Autodesk Fusion 360 part; units mm, degrees
(part 3 of 4)
  spline S213 degree 3 poles (-242.4, 76) (-242.5104, 76) (-242.6, 76.0895) (-242.6, 76.2) knots 6 6 6 6 7 7 7 7
  line L339 (-242.6, 76.2) -> (-242.6, 89.8)
  spline S214 degree 3 poles (-242.6, 89.8) (-242.6, 89.9104) (-242.5104, 90) (-242.4, 90) knots 0 0 0 0 1 1 1 1
  line L340 (-242.4, 90) -> (-228.8, 90)
  spline S215 degree 3 poles (-228.8, 90) (-228.6896, 90) (-228.6, 89.9104) (-228.6, 89.8) knots 2 2 2 2 3 3 3 3
  line L341 (-228.6, 89.8) -> (-228.6, 76.2)
  spline S216 degree 3 poles (-228.6, 76.2) (-228.6, 76.0895) (-228.6896, 76) (-228.8, 76) knots 4 4 4 4 5 5 5 5
  line L342 (-228.8, 76) -> (-242.4, 76)
  spline S217 degree 3 poles (-240.705, 70.95) (-240.5946, 70.95) (-240.505, 70.8604) (-240.505, 70.75) knots 6 6 6 6 7 7 7 7
  line L343 (-240.505, 70.75) -> (-240.505, 57.15)
  spline S218 degree 3 poles (-240.505, 57.15) (-240.505, 57.0395) (-240.5946, 56.95) (-240.705, 56.95) knots 0 0 0 0 1 1 1 1
  line L344 (-240.705, 56.95) -> (-254.3051, 56.95)
  spline S219 degree 3 poles (-254.3051, 56.95) (-254.4155, 56.95) (-254.5051, 57.0395) (-254.5051, 57.15) knots 2 2 2 2 3 3 3 3
  line L345 (-254.5051, 57.15) -> (-254.5051, 70.75)
  spline S220 degree 3 poles (-254.5051, 70.75) (-254.5051, 70.8604) (-254.4155, 70.95) (-254.3051, 70.95) knots 4 4 4 4 5 5 5 5
  line L346 (-254.3051, 70.95) -> (-240.705, 70.95)
  spline S221 degree 3 poles (-157.3601, 70.95) (-157.2497, 70.95) (-157.1601, 70.8604) (-157.1601, 70.75) knots 6 6 6 6 7 7 7 7
  line L347 (-157.1601, 70.75) -> (-157.1601, 57.15)
  spline S222 degree 3 poles (-157.1601, 57.15) (-157.1601, 57.0395) (-157.2497, 56.95) (-157.3601, 56.95) knots 0 0 0 0 1 1 1 1
  line L348 (-157.3601, 56.95) -> (-170.9601, 56.95)
  spline S223 degree 3 poles (-170.9601, 56.95) (-171.0705, 56.95) (-171.1601, 57.0395) (-171.1601, 57.15) knots 2 2 2 2 3 3 3 3
  line L349 (-171.1601, 57.15) -> (-171.1601, 70.75)
  spline S224 degree 3 poles (-171.1601, 70.75) (-171.1601, 70.8604) (-171.0705, 70.95) (-170.9601, 70.95) knots 4 4 4 4 5 5 5 5
  line L350 (-170.9601, 70.95) -> (-157.3601, 70.95)
  spline S225 degree 3 poles (-180.6801, 51.7) (-180.6801, 51.8104) (-180.5905, 51.9) (-180.4801, 51.9) knots 6 6 6 6 7 7 7 7
  line L351 (-180.4801, 51.9) -> (-166.8801, 51.9)
  spline S226 degree 3 poles (-166.8801, 51.9) (-166.7697, 51.9) (-166.6801, 51.8104) (-166.6801, 51.7) knots 0 0 0 0 1 1 1 1
  line L352 (-166.6801, 51.7) -> (-166.6801, 38.1)
  spline S227 degree 3 poles (-166.6801, 38.1) (-166.6801, 37.9895) (-166.7697, 37.9) (-166.8801, 37.9) knots 2 2 2 2 3 3 3 3
  line L353 (-166.8801, 37.9) -> (-180.4801, 37.9)
  spline S228 degree 3 poles (-180.4801, 37.9) (-180.5905, 37.9) (-180.6801, 37.9895) (-180.6801, 38.1) knots 4 4 4 4 5 5 5 5
  line L354 (-180.6801, 38.1) -> (-180.6801, 51.7)
  spline S229 degree 3 poles (-152.6, 13.8) (-152.4896, 13.8) (-152.4, 13.7104) (-152.4, 13.6) knots 6 6 6 6 7 7 7 7
  line L355 (-152.4, 13.6) -> (-152.4, 0)
  spline S230 degree 3 poles (-152.4, 0) (-152.4, -0.1105) (-152.4896, -0.2) (-152.6, -0.2) knots 0 0 0 0 1 1 1 1
  line L356 (-152.6, -0.2) -> (-166.2, -0.2)
  spline S231 degree 3 poles (-166.2, -0.2) (-166.3104, -0.2) (-166.4, -0.1105) (-166.4, 0) knots 2 2 2 2 3 3 3 3
  line L357 (-166.4, 0) -> (-166.4, 13.6)
  spline S232 degree 3 poles (-166.4, 13.6) (-166.4, 13.7104) (-166.3104, 13.8) (-166.2, 13.8) knots 4 4 4 4 5 5 5 5
  line L358 (-166.2, 13.8) -> (-152.6, 13.8)
  line L359 (-156.68, 32.85) -> (-143.0802, 32.85)
  spline S233 degree 3 poles (-143.0802, 32.85) (-142.9696, 32.85) (-142.88, 32.7604) (-142.88, 32.65) knots 7 7 7 7 8 8 8 8
  line L360 (-142.88, 32.65) -> (-142.88, 19.05)
  spline S234 degree 3 poles (-142.88, 19.05) (-142.88, 18.9395) (-142.9696, 18.85) (-143.0802, 18.85) knots 1 1 1 1 2 2 2 2
  line L361 (-143.0802, 18.85) -> (-156.68, 18.85)
  spline S235 degree 3 poles (-156.68, 18.85) (-156.7906, 18.85) (-156.88, 18.9395) (-156.88, 19.05) knots 3 3 3 3 4 4 4 4
  line L362 (-156.88, 19.05) -> (-156.88, 32.65)
  spline S236 degree 3 poles (-156.88, 32.65) (-156.88, 32.7604) (-156.7906, 32.85) (-156.68, 32.85) knots 5 5 5 5 6 6 6 6
  line L363 (-118.58, 32.85) -> (-104.9802, 32.85)
  spline S237 degree 3 poles (-104.9802, 32.85) (-104.8696, 32.85) (-104.78, 32.7604) (-104.78, 32.65) knots 7 7 7 7 8 8 8 8
  line L364 (-104.78, 32.65) -> (-104.78, 19.05)
  spline S238 degree 3 poles (-104.78, 19.05) (-104.78, 18.9395) (-104.8696, 18.85) (-104.9802, 18.85) knots 1 1 1 1 2 2 2 2
  line L365 (-104.9802, 18.85) -> (-118.58, 18.85)
  spline S239 degree 3 poles (-118.58, 18.85) (-118.6906, 18.85) (-118.78, 18.9395) (-118.78, 19.05) knots 3 3 3 3 4 4 4 4
  line L366 (-118.78, 19.05) -> (-118.78, 32.65)
  spline S240 degree 3 poles (-118.78, 32.65) (-118.78, 32.7604) (-118.6906, 32.85) (-118.58, 32.85) knots 5 5 5 5 6 6 6 6
  line L367 (-175.73, 32.85) -> (-162.1302, 32.85)
  spline S241 degree 3 poles (-162.1302, 32.85) (-162.0196, 32.85) (-161.93, 32.7604) (-161.93, 32.65) knots 7 7 7 7 8 8 8 8
  line L368 (-161.93, 32.65) -> (-161.93, 19.05)
  spline S242 degree 3 poles (-161.93, 19.05) (-161.93, 18.9395) (-162.0196, 18.85) (-162.1302, 18.85) knots 1 1 1 1 2 2 2 2
  line L369 (-162.1302, 18.85) -> (-175.73, 18.85)
  spline S243 degree 3 poles (-175.73, 18.85) (-175.8406, 18.85) (-175.93, 18.9395) (-175.93, 19.05) knots 3 3 3 3 4 4 4 4
  line L370 (-175.93, 19.05) -> (-175.93, 32.65)
  spline S244 degree 3 poles (-175.93, 32.65) (-175.93, 32.7604) (-175.8406, 32.85) (-175.73, 32.85) knots 5 5 5 5 6 6 6 6
  line L371 (-99.53, 32.85) -> (-85.9302, 32.85)
  spline S245 degree 3 poles (-85.9302, 32.85) (-85.8196, 32.85) (-85.73, 32.7604) (-85.73, 32.65) knots 7 7 7 7 8 8 8 8
  line L372 (-85.73, 32.65) -> (-85.73, 19.05)
  spline S246 degree 3 poles (-85.73, 19.05) (-85.73, 18.9395) (-85.8196, 18.85) (-85.9302, 18.85) knots 1 1 1 1 2 2 2 2
  line L373 (-85.9302, 18.85) -> (-99.53, 18.85)
  spline S247 degree 3 poles (-99.53, 18.85) (-99.6406, 18.85) (-99.73, 18.9395) (-99.73, 19.05) knots 3 3 3 3 4 4 4 4
  line L374 (-99.73, 19.05) -> (-99.73, 32.65)
  spline S248 degree 3 poles (-99.73, 32.65) (-99.73, 32.7604) (-99.6406, 32.85) (-99.53, 32.85) knots 5 5 5 5 6 6 6 6
  spline S249 degree 3 poles (-138.3101, 70.95) (-138.1997, 70.95) (-138.1101, 70.8604) (-138.1101, 70.75) knots 6 6 6 6 7 7 7 7
  line L375 (-138.1101, 70.75) -> (-138.1101, 57.15)
  spline S250 degree 3 poles (-138.1101, 57.15) (-138.1101, 57.0395) (-138.1997, 56.95) (-138.3101, 56.95) knots 0 0 0 0 1 1 1 1
  line L376 (-138.3101, 56.95) -> (-151.9101, 56.95)
  spline S251 degree 3 poles (-151.9101, 56.95) (-152.0205, 56.95) (-152.1101, 57.0395) (-152.1101, 57.15) knots 2 2 2 2 3 3 3 3
  line L377 (-152.1101, 57.15) -> (-152.1101, 70.75)
  spline S252 degree 3 poles (-152.1101, 70.75) (-152.1101, 70.8604) (-152.0205, 70.95) (-151.9101, 70.95) knots 4 4 4 4 5 5 5 5
  line L378 (-151.9101, 70.95) -> (-138.3101, 70.95)
  spline S253 degree 3 poles (-52.5801, 51.9) (-52.4697, 51.9) (-52.3801, 51.8104) (-52.3801, 51.7) knots 6 6 6 6 7 7 7 7
  line L379 (-52.3801, 51.7) -> (-52.3801, 38.1)
  spline S254 degree 3 poles (-52.3801, 38.1) (-52.3801, 37.9895) (-52.4697, 37.9) (-52.5801, 37.9) knots 0 0 0 0 1 1 1 1
  line L380 (-52.5801, 37.9) -> (-66.1801, 37.9)
  spline S255 degree 3 poles (-66.1801, 37.9) (-66.2905, 37.9) (-66.3801, 37.9895) (-66.3801, 38.1) knots 2 2 2 2 3 3 3 3
  line L381 (-66.3801, 38.1) -> (-66.3801, 51.7)
  spline S256 degree 3 poles (-66.3801, 51.7) (-66.3801, 51.8104) (-66.2905, 51.9) (-66.1801, 51.9) knots 4 4 4 4 5 5 5 5
  line L382 (-66.1801, 51.9) -> (-52.5801, 51.9)
  line L383 (-80.48, 32.85) -> (-66.8802, 32.85)
  spline S257 degree 3 poles (-66.8802, 32.85) (-66.7696, 32.85) (-66.68, 32.7604) (-66.68, 32.65) knots 7 7 7 7 8 8 8 8
  line L384 (-66.68, 32.65) -> (-66.68, 19.05)
  spline S258 degree 3 poles (-66.68, 19.05) (-66.68, 18.9395) (-66.7696, 18.85) (-66.8802, 18.85) knots 1 1 1 1 2 2 2 2
  line L385 (-66.8802, 18.85) -> (-80.48, 18.85)
  spline S259 degree 3 poles (-80.48, 18.85) (-80.5906, 18.85) (-80.68, 18.9395) (-80.68, 19.05) knots 3 3 3 3 4 4 4 4
  line L386 (-80.68, 19.05) -> (-80.68, 32.65)
  spline S260 degree 3 poles (-80.68, 32.65) (-80.68, 32.7604) (-80.5906, 32.85) (-80.48, 32.85) knots 5 5 5 5 6 6 6 6
  spline S261 degree 3 poles (-114.5, 13.8) (-114.3896, 13.8) (-114.3, 13.7104) (-114.3, 13.6) knots 6 6 6 6 7 7 7 7
  line L387 (-114.3, 13.6) -> (-114.3, 0)
  spline S262 degree 3 poles (-114.3, 0) (-114.3, -0.1105) (-114.3896, -0.2) (-114.5, -0.2) knots 0 0 0 0 1 1 1 1
  line L388 (-114.5, -0.2) -> (-128.1, -0.2)
  spline S263 degree 3 poles (-128.1, -0.2) (-128.2104, -0.2) (-128.3, -0.1105) (-128.3, 0) knots 2 2 2 2 3 3 3 3
  line L389 (-128.3, 0) -> (-128.3, 13.6)
  spline S264 degree 3 poles (-128.3, 13.6) (-128.3, 13.7104) (-128.2104, 13.8) (-128.1, 13.8) knots 4 4 4 4 5 5 5 5
  line L390 (-128.1, 13.8) -> (-114.5, 13.8)
  spline S265 degree 3 poles (-214.03, 32.65) (-214.03, 32.7604) (-213.9406, 32.85) (-213.83, 32.85) knots 6 6 6 6 7 7 7 7
  line L391 (-213.83, 32.85) -> (-200.2302, 32.85)
  spline S266 degree 3 poles (-200.2302, 32.85) (-200.1196, 32.85) (-200.03, 32.7604) (-200.03, 32.65) knots 0 0 0 0 1 1 1 1
  line L392 (-200.03, 32.65) -> (-200.03, 19.05)
  spline S267 degree 3 poles (-200.03, 19.05) (-200.03, 18.9395) (-200.1196, 18.85) (-200.2302, 18.85) knots 2 2 2 2 3 3 3 3
  line L393 (-200.2302, 18.85) -> (-213.83, 18.85)
  spline S268 degree 3 poles (-213.83, 18.85) (-213.9406, 18.85) (-214.03, 18.9395) (-214.03, 19.05) knots 4 4 4 4 5 5 5 5
  line L394 (-214.03, 19.05) -> (-214.03, 32.65)
  spline S269 degree 3 poles (-171.65, 13.8) (-171.5396, 13.8) (-171.45, 13.7104) (-171.45, 13.6) knots 6 6 6 6 7 7 7 7
  line L395 (-171.45, 13.6) -> (-171.45, 0)
  spline S270 degree 3 poles (-171.45, 0) (-171.45, -0.1105) (-171.5396, -0.2) (-171.65, -0.2) knots 0 0 0 0 1 1 1 1
  line L396 (-171.65, -0.2) -> (-185.25, -0.2)
  spline S271 degree 3 poles (-185.25, -0.2) (-185.3604, -0.2) (-185.45, -0.1105) (-185.45, 0) knots 2 2 2 2 3 3 3 3
  line L397 (-185.45, 0) -> (-185.45, 13.6)
  spline S272 degree 3 poles (-185.45, 13.6) (-185.45, 13.7104) (-185.3604, 13.8) (-185.25, 13.8) knots 4 4 4 4 5 5 5 5
  line L398 (-185.25, 13.8) -> (-171.65, 13.8)
  arc A8 (13, 95) -> (5, 103) centre (5, 95) ccw
  line L399 (5, 103) -> (-304.75, 103)
  arc A9 (-304.75, 103) -> (-312.75, 95) centre (-304.75, 95) ccw
  line L400 (-312.75, 95) -> (-312.75, -5.2)
  arc A10 (-312.75, -5.2) -> (-304.75, -13.2) centre (-304.75, -5.2) ccw
  line L401 (-304.75, -13.2) -> (5, -13.2)
  arc A11 (5, -13.2) -> (13, -5.2) centre (5, -5.2) ccw
  line L402 (13, -5.2) -> (13, 95)
  line L403 (3, -3.2) -> (-302.75, -3.2)
  line L404 (-302.75, -3.2) -> (-302.75, 93)
  line L405 (-302.75, 93) -> (3, 93)
  line L406 (3, 93) -> (3, -3.2)
  dimension "d354" = 3
  dimension "d355" = 3
  dimension "d356" = 3
  dimension "d358" = 3
  constraint horizontal L403
  constraint vertical L404
  constraint horizontal L405
  constraint vertical L406
  measures "d354" distance of L323 L404
  measures "d355" distance of L326 L403
  measures "d356" distance of L45 L405
  measures "d358" distance of L33 L406
extrude "Extrude2" add sketch "led-plate" along normal blind 3 separate body contours A8 L399 A9 L400 A10 L401 A11 L402 makes body 2 in component "led-plate"
sketch "top-plate" plane through (0, 0, 4.5) normal (0, 0, 1) x (-1, 0, 0) in component "top-plate"
  circle A0 centre (-228.8125, 98) radius 1
  circle A1 centre (-70.9375, 98) radius 1
  circle A2 centre (-70.9375, -8.2) radius 1
  circle A3 centre (-307.75, -8.2) radius 1
  circle A4 centre (-307.75, 98) radius 1
  circle A5 centre (8, 98) radius 1
  circle A6 centre (-228.8125, -8.2) radius 1
  circle A7 centre (8, -8.2) radius 1
  arc A8 (13, 95) -> (5, 103) centre (5, 95) ccw
  line L0 (5, 103) -> (-304.75, 103)
  arc A9 (-304.75, 103) -> (-312.75, 95) centre (-304.75, 95) ccw
  line L1 (-312.75, 95) -> (-312.75, -5.2)
  arc A10 (-312.75, -5.2) -> (-304.75, -13.2) centre (-304.75, -5.2) ccw
  line L2 (-304.75, -13.2) -> (5, -13.2)
  arc A11 (5, -13.2) -> (13, -5.2) centre (5, -5.2) ccw
  line L3 (13, -5.2) -> (13, 95)
  line L4 (8, -8.2) -> (8, 98) construction
  line L5 (8, 10.7161) -> (8, 79.0839)
  line L6 (13, -5.2) -> (13, 4.8)
  line L7 (13, 95) -> (13, 85)
  arc A12 (8, 10.7161) -> (10.5, 7.758) centre (11, 10.7161) ccw
  arc A13 (10.5, 82.042) -> (13, 85) centre (10, 85) ccw
  arc A14 (13, 4.8) -> (10.5, 7.758) centre (10, 4.8) ccw
  arc A15 (10.5, 82.042) -> (8, 79.0839) centre (11, 79.0839) ccw
  line L8 (-307.75, -8.2) -> (-307.75, 98) construction
  line L9 (-312.75, -5.2) -> (-312.75, 4.8)
  line L10 (-312.75, 95) -> (-312.75, 85)
  line L11 (-307.75, 79.0839) -> (-307.75, 10.7161)
  arc A16 (-310.25, 7.758) -> (-312.75, 4.8) centre (-309.75, 4.8) ccw
  arc A17 (-310.25, 7.758) -> (-307.75, 10.7161) centre (-310.75, 10.7161) ccw
  arc A18 (-307.75, 79.0839) -> (-310.25, 82.042) centre (-310.75, 79.0839) ccw
  arc A19 (-312.75, 85) -> (-310.25, 82.042) centre (-309.75, 85) ccw
  circle A20 centre (-307.75, 98) radius 1
  circle A21 centre (8, 98) radius 1
  circle A22 centre (-307.75, -8.2) radius 1
  circle A23 centre (-228.8125, -8.2) radius 1
  line L12 (-302.75, 93) -> (3, 93)
  line L13 (3, 93) -> (3, -3.2)
  line L14 (3, -3.2) -> (-302.75, -3.2)
  line L15 (-302.75, -3.2) -> (-302.75, 93)
  circle A24 centre (-228.8125, 98) radius 1
  circle A25 centre (-70.9375, 98) radius 1
  circle A26 centre (-70.9375, -8.2) radius 1
  circle A27 centre (8, -8.2) radius 1
  line L16 (13, -5.2) -> (13, 95)
  arc A28 (13, 95) -> (5, 103) centre (5, 95) ccw
  line L17 (5, 103) -> (-304.75, 103)
  arc A29 (-304.75, 103) -> (-312.75, 95) centre (-304.75, 95) ccw
  line L18 (-312.75, 95) -> (-312.75, -5.2)
  arc A30 (-312.75, -5.2) -> (-304.75, -13.2) centre (-304.75, -5.2) ccw
  line L19 (-304.75, -13.2) -> (5, -13.2)
  arc A31 (5, -13.2) -> (13, -5.2) centre (5, -5.2) ccw
  dimension "d322" = 3
  dimension "d332" = 10
  constraint coincident A7.centre L4.start
  constraint coincident A5.centre L4.end
  constraint coincident L4 L5.start
  constraint tangent L4 A12
  constraint tangent L7 A13
  constraint tangent A12 A14
  constraint tangent L6 A14
  constraint equal A13 A14
  constraint coincident L4 L5
  constraint tangent L5 A15
  constraint tangent A13 A15
  constraint equal A12 A14
  constraint vertical L7
  constraint vertical L6
  constraint equal L6 L7
  constraint coincident A11.end L3.start
  constraint coincident A3.centre L8.start
  constraint coincident A4.centre L8.end
  constraint parallel L1 L9
  constraint parallel L1 L10
  constraint tangent L9 A16
  constraint tangent A16 A17
  constraint tangent L11 A17
  constraint equal A13 A15
  constraint equal A14 A16
  constraint tangent L11 A18
  constraint tangent A18 A19
  constraint tangent L10 A19
  constraint equal A18 A19
  constraint equal A17 A18
  constraint equal L9 L10
  constraint coincident A9.end L1.start
  constraint equal L6 L9
  constraint coincident L1.end A10.start
  constraint coincident A8.start L3.end
  constraint coincident L8 L11.start
  constraint coincident L8 L11.end
  constraint equal A16 A17
  measures "d322" radius of A13
  measures "d332" distance of L6.end A11.end
extrude "Extrude2'" add sketch "top-plate" along normal blind 3 separate body contours A8 L0 A9 L1 A10 L2 A11 L3 L5 L6 L7 A12 A13 A14 A15 L9 L10 L11 A16 A17 A18 A19 L16 A28 L17 A29 L18 A30 L19 A31 makes body 3 in component "top-plate"
sketch "Sketch1" plane through (0, 0, 0) normal (0, 0, -1) x (1, 0, 0) in component "usb-plate"
  spline S0 degree 3 poles (57.35, 13.8) (57.2396, 13.8) (57.15, 13.7104) (57.15, 13.6) knots 6 6 6 6 7 7 7 7
  line L0 (57.35, 13.8) -> (70.95, 13.8)
  spline S1 degree 3 poles (71.15, 13.6) (71.15, 13.7104) (71.0604, 13.8) (70.95, 13.8) knots 4 4 4 4 5 5 5 5
  line L1 (71.15, 13.6) -> (71.15, 0)
  spline S2 degree 3 poles (70.95, -0.2) (71.0604, -0.2) (71.15, -0.1105) (71.15, 0) knots 2 2 2 2 3 3 3 3
  line L2 (70.95, -0.2) -> (57.35, -0.2)
  spline S3 degree 3 poles (57.15, 0) (57.15, -0.1105) (57.2396, -0.2) (57.35, -0.2) knots 0 0 0 0 1 1 1 1
  line L3 (57.15, 0) -> (57.15, 13.6)
  spline S4 degree 3 poles (42.58, 32.65) (42.58, 32.7604) (42.4906, 32.85) (42.38, 32.85) knots 6 6 6 6 7 7 7 7
  line L4 (42.58, 32.65) -> (42.58, 19.05)
  spline S5 degree 3 poles (42.38, 18.85) (42.4906, 18.85) (42.58, 18.9395) (42.58, 19.05) knots 4 4 4 4 5 5 5 5
  line L5 (42.38, 18.85) -> (28.7802, 18.85)
  spline S6 degree 3 poles (28.58, 19.05) (28.58, 18.9395) (28.6696, 18.85) (28.7802, 18.85) knots 2 2 2 2 3 3 3 3
  line L6 (28.58, 19.05) -> (28.58, 32.65)
  spline S7 degree 3 poles (28.7802, 32.85) (28.6696, 32.85) (28.58, 32.7604) (28.58, 32.65) knots 0 0 0 0 1 1 1 1
  line L7 (28.7802, 32.85) -> (42.38, 32.85)
  circle A0 centre (228.8125, -8.2) radius 1
  circle A1 centre (307.75, -8.2) radius 1
  circle A2 centre (307.75, 98) radius 1
  circle A3 centre (-8, 98) radius 1
  circle A4 centre (-8, -8.2) radius 1
  circle A5 centre (70.9375, -8.2) radius 1
  circle A6 centre (70.9375, 98) radius 1
  circle A7 centre (228.8125, 98) radius 1
  line L8 (18.5501, 18.85) -> (4.9501, 18.85)
  spline S8 degree 3 poles (4.7501, 19.05) (4.7501, 18.9395) (4.8397, 18.85) (4.9501, 18.85) knots 5 5 5 5 6 6 6 6
  line L9 (4.7501, 19.05) -> (4.7501, 32.65)
  spline S9 degree 3 poles (4.9501, 32.85) (4.8397, 32.85) (4.7501, 32.7604) (4.7501, 32.65) knots 3 3 3 3 4 4 4 4
  line L10 (4.9501, 32.85) -> (18.5501, 32.85)
  spline S10 degree 3 poles (18.7501, 32.65) (18.7501, 32.7604) (18.6605, 32.85) (18.5501, 32.85) knots 1 1 1 1 2 2 2 2
  line L11 (18.7501, 32.65) -> (18.7501, 19.05)
  spline S11 degree 3 poles (18.5501, 18.85) (18.6605, 18.85) (18.7501, 18.9395) (18.7501, 19.05) knots 7 7 7 7 8 8 8 8
  spline S12 degree 3 poles (63.7501, 76) (63.8605, 76) (63.9501, 76.0895) (63.9501, 76.2) knots 6 6 6 6 7 7 7 7
  line L12 (63.7501, 76) -> (50.1501, 76)
  spline S13 degree 3 poles (49.9501, 76.2) (49.9501, 76.0895) (50.0397, 76) (50.1501, 76) knots 4 4 4 4 5 5 5 5
  line L13 (49.9501, 76.2) -> (49.9501, 89.8)
  spline S14 degree 3 poles (50.1501, 90) (50.0397, 90) (49.9501, 89.9104) (49.9501, 89.8) knots 2 2 2 2 3 3 3 3
  line L14 (50.1501, 90) -> (63.7501, 90)
  spline S15 degree 3 poles (63.9501, 89.8) (63.9501, 89.9104) (63.8605, 90) (63.7501, 90) knots 0 0 0 0 1 1 1 1
  line L15 (63.9501, 89.8) -> (63.9501, 76.2)
  spline S16 degree 3 poles (39.95, 76) (40.0604, 76) (40.15, 76.0895) (40.15, 76.2) knots 6 6 6 6 7 7 7 7
  line L16 (39.95, 76) -> (26.35, 76)
  spline S17 degree 3 poles (26.15, 76.2) (26.15, 76.0895) (26.2396, 76) (26.35, 76) knots 4 4 4 4 5 5 5 5
  line L17 (26.15, 76.2) -> (26.15, 89.8)
  spline S18 degree 3 poles (26.35, 90) (26.2396, 90) (26.15, 89.9104) (26.15, 89.8) knots 2 2 2 2 3 3 3 3
  line L18 (26.35, 90) -> (39.95, 90)
  spline S19 degree 3 poles (40.15, 89.8) (40.15, 89.9104) (40.0604, 90) (39.95, 90) knots 0 0 0 0 1 1 1 1
  line L19 (40.15, 89.8) -> (40.15, 76.2)
  spline S20 degree 3 poles (33.5301, 51.9) (33.4197, 51.9) (33.3301, 51.8104) (33.3301, 51.7) knots 6 6 6 6 7 7 7 7
  line L20 (33.5301, 51.9) -> (47.1301, 51.9)
  spline S21 degree 3 poles (47.3301, 51.7) (47.3301, 51.8104) (47.2405, 51.9) (47.1301, 51.9) knots 4 4 4 4 5 5 5 5
  line L21 (47.3301, 51.7) -> (47.3301, 38.1)
  spline S22 degree 3 poles (47.1301, 37.9) (47.2405, 37.9) (47.3301, 37.9895) (47.3301, 38.1) knots 2 2 2 2 3 3 3 3
  line L22 (47.1301, 37.9) -> (33.5301, 37.9)
  spline S23 degree 3 poles (33.3301, 38.1) (33.3301, 37.9895) (33.4197, 37.9) (33.5301, 37.9) knots 0 0 0 0 1 1 1 1
  line L23 (33.3301, 38.1) -> (33.3301, 51.7)
  line L24 (20.9402, 37.9) -> (7.3401, 37.9)
  spline S24 degree 3 poles (7.1401, 38.1) (7.1401, 37.9895) (7.2297, 37.9) (7.3401, 37.9) knots 5 5 5 5 6 6 6 6
  line L25 (7.1401, 38.1) -> (7.1401, 51.7)
  spline S25 degree 3 poles (7.3401, 51.9) (7.2297, 51.9) (7.1401, 51.8104) (7.1401, 51.7) knots 3 3 3 3 4 4 4 4
  line L26 (7.3401, 51.9) -> (20.9402, 51.9)
  spline S26 degree 3 poles (21.1401, 51.7) (21.1401, 51.8104) (21.0506, 51.9) (20.9402, 51.9) knots 1 1 1 1 2 2 2 2
  line L27 (21.1401, 51.7) -> (21.1401, 38.1)
  spline S27 degree 3 poles (20.9402, 37.9) (21.0506, 37.9) (21.1401, 37.9895) (21.1401, 38.1) knots 7 7 7 7 8 8 8 8
  spline S28 degree 3 poles (76.4, 13.8) (76.2896, 13.8) (76.2, 13.7104) (76.2, 13.6) knots 6 6 6 6 7 7 7 7
  line L28 (76.4, 13.8) -> (90, 13.8)
  spline S29 degree 3 poles (90.2, 13.6) (90.2, 13.7104) (90.1104, 13.8) (90, 13.8) knots 4 4 4 4 5 5 5 5
  line L29 (90.2, 13.6) -> (90.2, 0)
  spline S30 degree 3 poles (90, -0.2) (90.1104, -0.2) (90.2, -0.1105) (90.2, 0) knots 2 2 2 2 3 3 3 3
  line L30 (90, -0.2) -> (76.4, -0.2)
  spline S31 degree 3 poles (76.2, 0) (76.2, -0.1105) (76.2896, -0.2) (76.4, -0.2) knots 0 0 0 0 1 1 1 1
  line L31 (76.2, 0) -> (76.2, 13.6)
  line L32 (0.2, 13.8) -> (13.8, 13.8)
  spline S32 degree 3 poles (14, 13.6) (14, 13.7104) (13.9104, 13.8) (13.8, 13.8) knots 5 5 5 5 6 6 6 6
  line L33 (14, 13.6) -> (14, 0)
  spline S33 degree 3 poles (13.8, -0.2) (13.9104, -0.2) (14, -0.1105) (14, 0) knots 3 3 3 3 4 4 4 4
  line L34 (13.8, -0.2) -> (0.2, -0.2)
  spline S34 degree 3 poles (0, 0) (0, -0.1105) (0.0896, -0.2) (0.2, -0.2) knots 1 1 1 1 2 2 2 2
  line L35 (0, 0) -> (0, 13.6)
  spline S35 degree 3 poles (0.2, 13.8) (0.0896, 13.8) (0, 13.7104) (0, 13.6) knots 7 7 7 7 8 8 8 8
  spline S36 degree 3 poles (209.0601, 56.95) (209.1705, 56.95) (209.2601, 57.0395) (209.2601, 57.15) knots 6 6 6 6 7 7 7 7
  line L36 (209.0601, 56.95) -> (195.4601, 56.95)
  spline S37 degree 3 poles (195.2601, 57.15) (195.2601, 57.0395) (195.3497, 56.95) (195.4601, 56.95) knots 4 4 4 4 5 5 5 5
  line L37 (195.2601, 57.15) -> (195.2601, 70.75)
  spline S38 degree 3 poles (195.4601, 70.95) (195.3497, 70.95) (195.2601, 70.8604) (195.2601, 70.75) knots 2 2 2 2 3 3 3 3
  line L38 (195.4601, 70.95) -> (209.0601, 70.95)
  spline S39 degree 3 poles (209.2601, 70.75) (209.2601, 70.8604) (209.1705, 70.95) (209.0601, 70.95) knots 0 0 0 0 1 1 1 1
  line L39 (209.2601, 70.75) -> (209.2601, 57.15)
  spline S40 degree 3 poles (190.0101, 56.95) (190.1205, 56.95) (190.2101, 57.0395) (190.2101, 57.15) knots 6 6 6 6 7 7 7 7
  line L40 (190.0101, 56.95) -> (176.4101, 56.95)
  spline S41 degree 3 poles (176.2101, 57.15) (176.2101, 57.0395) (176.2997, 56.95) (176.4101, 56.95) knots 4 4 4 4 5 5 5 5
  line L41 (176.2101, 57.15) -> (176.2101, 70.75)
  spline S42 degree 3 poles (176.4101, 70.95) (176.2997, 70.95) (176.2101, 70.8604) (176.2101, 70.75) knots 2 2 2 2 3 3 3 3
  line L42 (176.4101, 70.95) -> (190.0101, 70.95)
  spline S43 degree 3 poles (190.2101, 70.75) (190.2101, 70.8604) (190.1205, 70.95) (190.0101, 70.95) knots 0 0 0 0 1 1 1 1
  line L43 (190.2101, 70.75) -> (190.2101, 57.15)
  spline S44 degree 3 poles (16.1501, 76) (16.2605, 76) (16.3501, 76.0895) (16.3501, 76.2) knots 6 6 6 6 7 7 7 7
  line L44 (16.1501, 76) -> (2.5501, 76)
  spline S45 degree 3 poles (2.3501, 76.2) (2.3501, 76.0895) (2.4396, 76) (2.5501, 76) knots 4 4 4 4 5 5 5 5
  line L45 (2.3501, 76.2) -> (2.3501, 89.8)
  spline S46 degree 3 poles (2.5501, 90) (2.4396, 90) (2.3501, 89.9104) (2.3501, 89.8) knots 2 2 2 2 3 3 3 3
  line L46 (2.5501, 90) -> (16.1501, 90)
  spline S47 degree 3 poles (16.3501, 89.8) (16.3501, 89.9104) (16.2605, 90) (16.1501, 90) knots 0 0 0 0 1 1 1 1
  line L47 (16.3501, 89.8) -> (16.3501, 76.2)
  spline S48 degree 3 poles (223.3576, 76) (223.468, 76) (223.5576, 76.0895) (223.5576, 76.2) knots 6 6 6 6 7 7 7 7
  line L48 (223.3576, 76) -> (209.7576, 76)
  spline S49 degree 3 poles (209.5576, 76.2) (209.5576, 76.0895) (209.6472, 76) (209.7576, 76) knots 4 4 4 4 5 5 5 5
  line L49 (209.5576, 76.2) -> (209.5576, 89.8)
  spline S50 degree 3 poles (209.7576, 90) (209.6472, 90) (209.5576, 89.9104) (209.5576, 89.8) knots 2 2 2 2 3 3 3 3
  line L50 (209.7576, 90) -> (223.3576, 90)
  spline S51 degree 3 poles (223.5576, 89.8) (223.5576, 89.9104) (223.468, 90) (223.3576, 90) knots 0 0 0 0 1 1 1 1
  line L51 (223.5576, 89.8) -> (223.5576, 76.2)
  spline S52 degree 3 poles (95.45, 13.8) (95.3396, 13.8) (95.25, 13.7104) (95.25, 13.6) knots 6 6 6 6 7 7 7 7
  line L52 (95.45, 13.8) -> (109.05, 13.8)
  spline S53 degree 3 poles (109.25, 13.6) (109.25, 13.7104) (109.1604, 13.8) (109.05, 13.8) knots 4 4 4 4 5 5 5 5
  line L53 (109.25, 13.6) -> (109.25, 0)
  spline S54 degree 3 poles (109.05, -0.2) (109.1604, -0.2) (109.25, -0.1105) (109.25, 0) knots 2 2 2 2 3 3 3 3
  line L54 (109.05, -0.2) -> (95.45, -0.2)
  spline S55 degree 3 poles (95.25, 0) (95.25, -0.1105) (95.3396, -0.2) (95.45, -0.2) knots 0 0 0 0 1 1 1 1
  line L55 (95.25, 0) -> (95.25, 13.6)
  spline S56 degree 3 poles (19.25, 13.8) (19.1396, 13.8) (19.05, 13.7104) (19.05, 13.6) knots 6 6 6 6 7 7 7 7
  line L56 (19.25, 13.8) -> (32.85, 13.8)
  spline S57 degree 3 poles (33.05, 13.6) (33.05, 13.7104) (32.9604, 13.8) (32.85, 13.8) knots 4 4 4 4 5 5 5 5
  line L57 (33.05, 13.6) -> (33.05, 0)
  spline S58 degree 3 poles (32.85, -0.2) (32.9604, -0.2) (33.05, -0.1105) (33.05, 0) knots 2 2 2 2 3 3 3 3
  line L58 (32.85, -0.2) -> (19.25, -0.2)
  spline S59 degree 3 poles (19.05, 0) (19.05, -0.1105) (19.1396, -0.2) (19.25, -0.2) knots 0 0 0 0 1 1 1 1
  line L59 (19.05, 0) -> (19.05, 13.6)
  spline S60 degree 3 poles (204.3, 76) (204.4104, 76) (204.5, 76.0895) (204.5, 76.2) knots 6 6 6 6 7 7 7 7
  line L60 (204.3, 76) -> (190.7, 76)
  spline S61 degree 3 poles (190.5, 76.2) (190.5, 76.0895) (190.5896, 76) (190.7, 76) knots 4 4 4 4 5 5 5 5
  line L61 (190.5, 76.2) -> (190.5, 89.8)
  spline S62 degree 3 poles (190.7, 90) (190.5896, 90) (190.5, 89.9104) (190.5, 89.8) knots 2 2 2 2 3 3 3 3
  line L62 (190.7, 90) -> (204.3, 90)
  spline S63 degree 3 poles (204.5, 89.8) (204.5, 89.9104) (204.4104, 90) (204.3, 90) knots 0 0 0 0 1 1 1 1
  line L63 (204.5, 89.8) -> (204.5, 76.2)
  line L64 (43.0601, 70.95) -> (56.6601, 70.95)
  spline S64 degree 3 poles (56.8601, 70.75) (56.8601, 70.8604) (56.7705, 70.95) (56.6601, 70.95) knots 5 5 5 5 6 6 6 6
  line L65 (56.8601, 70.75) -> (56.8601, 57.15)
  spline S65 degree 3 poles (56.6601, 56.95) (56.7705, 56.95) (56.8601, 57.0395) (56.8601, 57.15) knots 3 3 3 3 4 4 4 4
  line L66 (56.6601, 56.95) -> (43.0601, 56.95)
  spline S66 degree 3 poles (42.8601, 57.15) (42.8601, 57.0395) (42.9497, 56.95) (43.0601, 56.95) knots 1 1 1 1 2 2 2 2
  line L67 (42.8601, 57.15) -> (42.8601, 70.75)
  spline S67 degree 3 poles (43.0601, 70.95) (42.9497, 70.95) (42.8601, 70.8604) (42.8601, 70.75) knots 7 7 7 7 8 8 8 8
  spline S68 degree 3 poles (119.2601, 70.95) (119.1497, 70.95) (119.0601, 70.8604) (119.0601, 70.75) knots 6 6 6 6 7 7 7 7
  line L68 (119.2601, 70.95) -> (132.8601, 70.95)
  spline S69 degree 3 poles (133.0601, 70.75) (133.0601, 70.8604) (132.9705, 70.95) (132.8601, 70.95) knots 4 4 4 4 5 5 5 5
  line L69 (133.0601, 70.75) -> (133.0601, 57.15)
  spline S70 degree 3 poles (132.8601, 56.95) (132.9705, 56.95) (133.0601, 57.0395) (133.0601, 57.15) knots 2 2 2 2 3 3 3 3
  line L70 (132.8601, 56.95) -> (119.2601, 56.95)
  spline S71 degree 3 poles (119.0601, 57.15) (119.0601, 57.0395) (119.1497, 56.95) (119.2601, 56.95) knots 0 0 0 0 1 1 1 1
  line L71 (119.0601, 57.15) -> (119.0601, 70.75)
  spline S72 degree 3 poles (100.2101, 70.95) (100.0997, 70.95) (100.0101, 70.8604) (100.0101, 70.75) knots 6 6 6 6 7 7 7 7
  line L72 (100.2101, 70.95) -> (113.8101, 70.95)
  spline S73 degree 3 poles (114.0101, 70.75) (114.0101, 70.8604) (113.9205, 70.95) (113.8101, 70.95) knots 4 4 4 4 5 5 5 5
  line L73 (114.0101, 70.75) -> (114.0101, 57.15)
  spline S74 degree 3 poles (113.8101, 56.95) (113.9205, 56.95) (114.0101, 57.0395) (114.0101, 57.15) knots 2 2 2 2 3 3 3 3
  line L74 (113.8101, 56.95) -> (100.2101, 56.95)
  spline S75 degree 3 poles (100.0101, 57.15) (100.0101, 57.0395) (100.0997, 56.95) (100.2101, 56.95) knots 0 0 0 0 1 1 1 1
  line L75 (100.0101, 57.15) -> (100.0101, 70.75)
  spline S76 degree 3 poles (194.98, 32.65) (194.98, 32.7604) (194.8906, 32.85) (194.78, 32.85) knots 6 6 6 6 7 7 7 7
  line L76 (194.98, 32.65) -> (194.98, 19.05)
  spline S77 degree 3 poles (194.78, 18.85) (194.8906, 18.85) (194.98, 18.9395) (194.98, 19.05) knots 4 4 4 4 5 5 5 5
  line L77 (194.78, 18.85) -> (181.1802, 18.85)
  spline S78 degree 3 poles (180.98, 19.05) (180.98, 18.9395) (181.0696, 18.85) (181.1802, 18.85) knots 2 2 2 2 3 3 3 3
  line L78 (180.98, 19.05) -> (180.98, 32.65)
  spline S79 degree 3 poles (181.1802, 32.85) (181.0696, 32.85) (180.98, 32.7604) (180.98, 32.65) knots 0 0 0 0 1 1 1 1
  line L79 (181.1802, 32.85) -> (194.78, 32.85)
  spline S80 degree 3 poles (209.75, 13.8) (209.6396, 13.8) (209.55, 13.7104) (209.55, 13.6) knots 6 6 6 6 7 7 7 7
  line L80 (209.75, 13.8) -> (223.35, 13.8)
  spline S81 degree 3 poles (223.55, 13.6) (223.55, 13.7104) (223.4604, 13.8) (223.35, 13.8) knots 4 4 4 4 5 5 5 5
  line L81 (223.55, 13.6) -> (223.55, 0)
  spline S82 degree 3 poles (223.35, -0.2) (223.4604, -0.2) (223.55, -0.1105) (223.55, 0) knots 2 2 2 2 3 3 3 3
  line L82 (223.35, -0.2) -> (209.75, -0.2)
  spline S83 degree 3 poles (209.55, 0) (209.55, -0.1105) (209.6396, -0.2) (209.75, -0.2) knots 0 0 0 0 1 1 1 1
  line L83 (209.55, 0) -> (209.55, 13.6)
  spline S84 degree 3 poles (85.4301, 51.7) (85.4301, 51.8104) (85.3405, 51.9) (85.2301, 51.9) knots 6 6 6 6 7 7 7 7
  line L84 (85.4301, 51.7) -> (85.4301, 38.1)
  spline S85 degree 3 poles (85.2301, 37.9) (85.3405, 37.9) (85.4301, 37.9895) (85.4301, 38.1) knots 4 4 4 4 5 5 5 5
  line L85 (85.2301, 37.9) -> (71.6301, 37.9)
  spline S86 degree 3 poles (71.4301, 38.1) (71.4301, 37.9895) (71.5197, 37.9) (71.6301, 37.9) knots 2 2 2 2 3 3 3 3
  line L86 (71.4301, 38.1) -> (71.4301, 51.7)
  spline S87 degree 3 poles (71.6301, 51.9) (71.5197, 51.9) (71.4301, 51.8104) (71.4301, 51.7) knots 0 0 0 0 1 1 1 1
  line L87 (71.6301, 51.9) -> (85.2301, 51.9)
  spline S88 degree 3 poles (62.1101, 70.95) (61.9997, 70.95) (61.9101, 70.8604) (61.9101, 70.75) knots 6 6 6 6 7 7 7 7
  line L88 (62.1101, 70.95) -> (75.7101, 70.95)
  spline S89 degree 3 poles (75.9101, 70.75) (75.9101, 70.8604) (75.8205, 70.95) (75.7101, 70.95) knots 4 4 4 4 5 5 5 5
  line L89 (75.9101, 70.75) -> (75.9101, 57.15)
  spline S90 degree 3 poles (75.7101, 56.95) (75.8205, 56.95) (75.9101, 57.0395) (75.9101, 57.15) knots 2 2 2 2 3 3 3 3
  line L90 (75.7101, 56.95) -> (62.1101, 56.95)
  spline S91 degree 3 poles (61.9101, 57.15) (61.9101, 57.0395) (61.9997, 56.95) (62.1101, 56.95) knots 0 0 0 0 1 1 1 1
  line L91 (61.9101, 57.15) -> (61.9101, 70.75)
  spline S92 degree 3 poles (123.5301, 51.7) (123.5301, 51.8104) (123.4405, 51.9) (123.3301, 51.9) knots 6 6 6 6 7 7 7 7
  line L92 (123.5301, 51.7) -> (123.5301, 38.1)
  spline S93 degree 3 poles (123.3301, 37.9) (123.4405, 37.9) (123.5301, 37.9895) (123.5301, 38.1) knots 4 4 4 4 5 5 5 5
  line L93 (123.3301, 37.9) -> (109.7301, 37.9)
  spline S94 degree 3 poles (109.5301, 38.1) (109.5301, 37.9895) (109.6197, 37.9) (109.7301, 37.9) knots 2 2 2 2 3 3 3 3
  line L94 (109.5301, 38.1) -> (109.5301, 51.7)
  spline S95 degree 3 poles (109.7301, 51.9) (109.6197, 51.9) (109.5301, 51.8104) (109.5301, 51.7) knots 0 0 0 0 1 1 1 1
  line L95 (109.7301, 51.9) -> (123.3301, 51.9)
  spline S96 degree 3 poles (61.63, 32.65) (61.63, 32.7604) (61.5406, 32.85) (61.43, 32.85) knots 6 6 6 6 7 7 7 7
  line L96 (61.63, 32.65) -> (61.63, 19.05)
  spline S97 degree 3 poles (61.43, 18.85) (61.5406, 18.85) (61.63, 18.9395) (61.63, 19.05) knots 4 4 4 4 5 5 5 5
  line L97 (61.43, 18.85) -> (47.8302, 18.85)
  spline S98 degree 3 poles (47.63, 19.05) (47.63, 18.9395) (47.7196, 18.85) (47.8302, 18.85) knots 2 2 2 2 3 3 3 3
  line L98 (47.63, 19.05) -> (47.63, 32.65)
  spline S99 degree 3 poles (47.8302, 32.85) (47.7196, 32.85) (47.63, 32.7604) (47.63, 32.65) knots 0 0 0 0 1 1 1 1
  line L99 (47.8302, 32.85) -> (61.43, 32.85)
  line L100 (25.935, 68.18) -> (27.5857, 68.18)
  line L101 (27.5857, 68.18) -> (27.5857, 70.68)
  line L102 (27.5857, 70.68) -> (29.4108, 70.68)
  line L103 (29.4108, 70.68) -> (29.4108, 71.93)
  line L104 (29.4108, 71.93) -> (32.4108, 71.93)
  line L105 (32.4108, 71.93) -> (32.4108, 70.68)
  line L106 (32.4108, 70.68) -> (34.2358, 70.68)
  line L107 (34.2358, 70.68) -> (34.2358, 64.48)
  line L108 (34.2358, 64.48) -> (35.0607, 64.48)
  line L109 (35.0607, 64.48) -> (35.0607, 61.47)
  line L110 (35.0607, 61.47) -> (34.2358, 61.47)
  line L111 (34.2358, 61.47) -> (34.2358, 58.47)
  line L112 (34.2358, 58.47) -> (27.5857, 58.47)
  line L113 (27.5857, 58.47) -> (27.5857, 60.97)
  line L114 (27.5857, 60.97) -> (25.91, 60.97)
  line L115 (25.91, 60.97) -> (25.91, 57.15)
  spline S100 degree 3 poles (25.7101, 56.95) (25.8205, 56.95) (25.91, 57.0395) (25.91, 57.15) knots 22 22 22 22 23 23 23 23
  line L116 (25.7101, 56.95) -> (12.11, 56.95)
  spline S101 degree 3 poles (11.91, 57.15) (11.91, 57.0395) (11.9996, 56.95) (12.11, 56.95) knots 20 20 20 20 21 21 21 21
  line L117 (11.91, 57.15) -> (11.91, 60.97)
  line L118 (11.91, 60.97) -> (10.2347, 60.97)
  line L119 (10.2347, 60.97) -> (10.2347, 58.47)
  line L120 (10.2347, 58.47) -> (3.5848, 58.47)
  line L121 (3.5848, 58.47) -> (3.5848, 61.47)
  line L122 (3.5848, 61.47) -> (2.7597, 61.47)
  line L123 (2.7597, 61.47) -> (2.7597, 64.48)
  line L124 (2.7597, 64.48) -> (3.5848, 64.48)
  line L125 (3.5848, 64.48) -> (3.5848, 70.68)
  line L126 (3.5848, 70.68) -> (5.4097, 70.68)
  line L127 (5.4097, 70.68) -> (5.4097, 71.93)
  line L128 (5.4097, 71.93) -> (8.4097, 71.93)
  line L129 (8.4097, 71.93) -> (8.4097, 70.68)
  line L130 (8.4097, 70.68) -> (10.2345, 70.68)
  line L131 (10.2345, 70.68) -> (10.2345, 68.18)
  line L132 (10.2345, 68.18) -> (11.91, 68.18)
  line L133 (11.91, 68.18) -> (11.91, 70.75)
  spline S102 degree 3 poles (12.11, 70.95) (11.9996, 70.95) (11.91, 70.8604) (11.91, 70.75) knots 2 2 2 2 3 3 3 3
  line L134 (12.11, 70.95) -> (25.735, 70.95)
  spline S103 degree 3 poles (25.935, 70.75) (25.935, 70.8604) (25.8456, 70.95) (25.735, 70.95) knots 0 0 0 0 1 1 1 1
  line L135 (25.935, 70.75) -> (25.935, 68.18)
  line L136 (182.6007, 80.52) -> (181.7758, 80.52)
  line L137 (181.7758, 80.52) -> (181.7758, 77.52)
  line L138 (181.7758, 77.52) -> (175.1254, 77.52)
  line L139 (175.1254, 77.52) -> (175.1254, 80.75)
  line L140 (175.1254, 80.75) -> (135.4501, 80.75)
  line L141 (135.4501, 80.75) -> (135.4501, 76.2)
  spline S104 degree 3 poles (135.2501, 76) (135.3606, 76) (135.4501, 76.0895) (135.4501, 76.2) knots 32 32 32 32 33 33 33 33
  line L142 (135.2501, 76) -> (121.6501, 76)
  spline S105 degree 3 poles (121.4501, 76.2) (121.4501, 76.0895) (121.5397, 76) (121.6501, 76) knots 30 30 30 30 31 31 31 31
  line L143 (121.4501, 76.2) -> (121.4501, 80.75)
  line L144 (121.4501, 80.75) -> (81.7747, 80.75)
  spline S106 degree 3 poles (81.7743, 77.52) (81.7743, 77.52) (81.7749, 80.75) (81.7747, 80.75) knots 27 27 27 27 28 28 28 28
  line L145 (81.7743, 77.52) -> (75.1244, 77.52)
  line L146 (75.1244, 77.52) -> (75.1244, 80.52)
  line L147 (75.1244, 80.52) -> (74.2993, 80.52)
  line L148 (74.2993, 80.52) -> (74.2993, 83.53)
  line L149 (74.2993, 83.53) -> (75.1244, 83.53)
  line L150 (75.1244, 83.53) -> (75.1244, 89.73)
  line L151 (75.1244, 89.73) -> (76.9495, 89.73)
  line L152 (76.9495, 89.73) -> (76.9495, 90)
  line L153 (76.9495, 90) -> (79.9495, 90)
  line L154 (79.9495, 90) -> (79.9495, 89.73)
  line L155 (79.9495, 89.73) -> (81.7745, 89.73)
  line L156 (81.7745, 89.73) -> (81.7745, 85.25)
  line L157 (81.7745, 85.25) -> (121.4501, 85.25)
  line L158 (121.4501, 85.25) -> (121.4501, 89.8)
  spline S107 degree 3 poles (121.6501, 90) (121.5397, 90) (121.4501, 89.9104) (121.4501, 89.8) knots 12 12 12 12 13 13 13 13
  line L159 (121.6501, 90) -> (135.2501, 90)
  spline S108 degree 3 poles (135.4501, 89.8) (135.4501, 89.9104) (135.3606, 90) (135.2501, 90) knots 10 10 10 10 11 11 11 11
  line L160 (135.4501, 89.8) -> (135.4501, 85.25)
  line L161 (135.4501, 85.25) -> (175.1256, 85.25)
  line L162 (175.1256, 85.25) -> (175.1256, 89.73)
  line L163 (175.1256, 89.73) -> (176.9508, 89.73)
  line L164 (176.9508, 89.73) -> (176.9508, 90)
  line L165 (176.9508, 90) -> (179.9508, 90)
  line L166 (179.9508, 90) -> (179.9508, 89.73)
  line L167 (179.9508, 89.73) -> (181.7758, 89.73)
  line L168 (181.7758, 89.73) -> (181.7758, 83.53)
  line L169 (181.7758, 83.53) -> (182.6007, 83.53)
  line L170 (182.6007, 83.53) -> (182.6007, 80.52)
  spline S109 degree 3 poles (38.3, 13.8) (38.1896, 13.8) (38.1, 13.7104) (38.1, 13.6) knots 6 6 6 6 7 7 7 7
  line L171 (38.3, 13.8) -> (51.9, 13.8)
  spline S110 degree 3 poles (52.1, 13.6) (52.1, 13.7104) (52.0104, 13.8) (51.9, 13.8) knots 4 4 4 4 5 5 5 5
  line L172 (52.1, 13.6) -> (52.1, 0)
  spline S111 degree 3 poles (51.9, -0.2) (52.0104, -0.2) (52.1, -0.1105) (52.1, 0) knots 2 2 2 2 3 3 3 3
  line L173 (51.9, -0.2) -> (38.3, -0.2)
  spline S112 degree 3 poles (38.1, 0) (38.1, -0.1105) (38.1896, -0.2) (38.3, -0.2) knots 0 0 0 0 1 1 1 1
  line L174 (38.1, 0) -> (38.1, 13.6)
  line L175 (124.0302, 32.85) -> (137.63, 32.85)
  spline S113 degree 3 poles (137.83, 32.65) (137.83, 32.7604) (137.7406, 32.85) (137.63, 32.85) knots 5 5 5 5 6 6 6 6
  line L176 (137.83, 32.65) -> (137.83, 19.05)
  spline S114 degree 3 poles (137.63, 18.85) (137.7406, 18.85) (137.83, 18.9395) (137.83, 19.05) knots 3 3 3 3 4 4 4 4
  line L177 (137.63, 18.85) -> (124.0302, 18.85)
  spline S115 degree 3 poles (123.83, 19.05) (123.83, 18.9395) (123.9196, 18.85) (124.0302, 18.85) knots 1 1 1 1 2 2 2 2
  line L178 (123.83, 19.05) -> (123.83, 32.65)
  spline S116 degree 3 poles (124.0302, 32.85) (123.9196, 32.85) (123.83, 32.7604) (123.83, 32.65) knots 7 7 7 7 8 8 8 8
  spline S117 degree 3 poles (104.4801, 51.7) (104.4801, 51.8104) (104.3905, 51.9) (104.2801, 51.9) knots 6 6 6 6 7 7 7 7
  line L179 (104.4801, 51.7) -> (104.4801, 38.1)
  spline S118 degree 3 poles (104.2801, 37.9) (104.3905, 37.9) (104.4801, 37.9895) (104.4801, 38.1) knots 4 4 4 4 5 5 5 5
  line L180 (104.2801, 37.9) -> (90.6801, 37.9)
  spline S119 degree 3 poles (90.4801, 38.1) (90.4801, 37.9895) (90.5697, 37.9) (90.6801, 37.9) knots 2 2 2 2 3 3 3 3
  line L181 (90.4801, 38.1) -> (90.4801, 51.7)
  spline S120 degree 3 poles (90.6801, 51.9) (90.5697, 51.9) (90.4801, 51.8104) (90.4801, 51.7) knots 0 0 0 0 1 1 1 1
  line L182 (90.6801, 51.9) -> (104.2801, 51.9)
  spline S121 degree 3 poles (81.1601, 70.95) (81.0497, 70.95) (80.9601, 70.8604) (80.9601, 70.75) knots 6 6 6 6 7 7 7 7
  line L183 (81.1601, 70.95) -> (94.7601, 70.95)
  spline S122 degree 3 poles (94.9601, 70.75) (94.9601, 70.8604) (94.8705, 70.95) (94.7601, 70.95) knots 4 4 4 4 5 5 5 5
  line L184 (94.9601, 70.75) -> (94.9601, 57.15)
  spline S123 degree 3 poles (94.7601, 56.95) (94.8705, 56.95) (94.9601, 57.0395) (94.9601, 57.15) knots 2 2 2 2 3 3 3 3
  line L185 (94.7601, 56.95) -> (81.1601, 56.95)
  spline S124 degree 3 poles (80.9601, 57.15) (80.9601, 57.0395) (81.0497, 56.95) (81.1601, 56.95) knots 0 0 0 0 1 1 1 1
  line L186 (80.9601, 57.15) -> (80.9601, 70.75)
  spline S125 degree 3 poles (190.7, 13.8) (190.5896, 13.8) (190.5, 13.7104) (190.5, 13.6) knots 6 6 6 6 7 7 7 7
  line L187 (190.7, 13.8) -> (204.3, 13.8)
  spline S126 degree 3 poles (204.5, 13.6) (204.5, 13.7104) (204.4104, 13.8) (204.3, 13.8) knots 4 4 4 4 5 5 5 5
  line L188 (204.5, 13.6) -> (204.5, 0)
  spline S127 degree 3 poles (204.3, -0.2) (204.4104, -0.2) (204.5, -0.1105) (204.5, 0) knots 2 2 2 2 3 3 3 3
  line L189 (204.3, -0.2) -> (190.7, -0.2)
  spline S128 degree 3 poles (190.5, 0) (190.5, -0.1105) (190.5896, -0.2) (190.7, -0.2) knots 0 0 0 0 1 1 1 1
  line L190 (190.5, 0) -> (190.5, 13.6)
  spline S129 degree 3 poles (142.5801, 51.7) (142.5801, 51.8104) (142.4905, 51.9) (142.3801, 51.9) knots 6 6 6 6 7 7 7 7
  line L191 (142.5801, 51.7) -> (142.5801, 38.1)
  spline S130 degree 3 poles (142.3801, 37.9) (142.4905, 37.9) (142.5801, 37.9895) (142.5801, 38.1) knots 4 4 4 4 5 5 5 5
  line L192 (142.3801, 37.9) -> (128.7801, 37.9)
  spline S131 degree 3 poles (128.5801, 38.1) (128.5801, 37.9895) (128.6697, 37.9) (128.7801, 37.9) knots 2 2 2 2 3 3 3 3
  line L193 (128.5801, 38.1) -> (128.5801, 51.7)
  spline S132 degree 3 poles (128.7801, 51.9) (128.6697, 51.9) (128.5801, 51.8104) (128.5801, 51.7) knots 0 0 0 0 1 1 1 1
  line L194 (128.7801, 51.9) -> (142.3801, 51.9)
  spline S133 degree 3 poles (185.9301, 51.9) (185.8197, 51.9) (185.7301, 51.8104) (185.7301, 51.7) knots 6 6 6 6 7 7 7 7
  line L195 (185.9301, 51.9) -> (199.5301, 51.9)
  spline S134 degree 3 poles (199.7301, 51.7) (199.7301, 51.8104) (199.6405, 51.9) (199.5301, 51.9) knots 4 4 4 4 5 5 5 5
  line L196 (199.7301, 51.7) -> (199.7301, 38.1)
  spline S135 degree 3 poles (199.5301, 37.9) (199.6405, 37.9) (199.7301, 37.9895) (199.7301, 38.1) knots 2 2 2 2 3 3 3 3
  line L197 (199.5301, 37.9) -> (185.9301, 37.9)
  spline S136 degree 3 poles (185.7301, 38.1) (185.7301, 37.9895) (185.8197, 37.9) (185.9301, 37.9) knots 0 0 0 0 1 1 1 1
  line L198 (185.7301, 38.1) -> (185.7301, 51.7)
  spline S137 degree 3 poles (204.9801, 51.9) (204.8697, 51.9) (204.7801, 51.8104) (204.7801, 51.7) knots 6 6 6 6 7 7 7 7
  line L199 (204.9801, 51.9) -> (218.5801, 51.9)
  spline S138 degree 3 poles (218.7801, 51.7) (218.7801, 51.8104) (218.6905, 51.9) (218.5801, 51.9) knots 4 4 4 4 5 5 5 5
  line L200 (218.7801, 51.7) -> (218.7801, 38.1)
  spline S139 degree 3 poles (218.5801, 37.9) (218.6905, 37.9) (218.7801, 37.9895) (218.7801, 38.1) knots 2 2 2 2 3 3 3 3
  line L201 (218.5801, 37.9) -> (204.9801, 37.9)
  spline S140 degree 3 poles (204.7801, 38.1) (204.7801, 37.9895) (204.8697, 37.9) (204.9801, 37.9) knots 0 0 0 0 1 1 1 1
  line L202 (204.7801, 38.1) -> (204.7801, 51.7)
  spline S141 degree 3 poles (133.55, 13.8) (133.4396, 13.8) (133.35, 13.7104) (133.35, 13.6) knots 6 6 6 6 7 7 7 7
  line L203 (133.55, 13.8) -> (147.15, 13.8)
  spline S142 degree 3 poles (147.35, 13.6) (147.35, 13.7104) (147.2604, 13.8) (147.15, 13.8) knots 4 4 4 4 5 5 5 5
  line L204 (147.35, 13.6) -> (147.35, 0)
  spline S143 degree 3 poles (147.15, -0.2) (147.2604, -0.2) (147.35, -0.1105) (147.35, 0) knots 2 2 2 2 3 3 3 3
  line L205 (147.15, -0.2) -> (133.55, -0.2)
  spline S144 degree 3 poles (133.35, 0) (133.35, -0.1105) (133.4396, -0.2) (133.55, -0.2) knots 0 0 0 0 1 1 1 1
  line L206 (133.35, 0) -> (133.35, 13.6)
  spline S145 degree 3 poles (161.6301, 51.7) (161.6301, 51.8104) (161.5405, 51.9) (161.4301, 51.9) knots 6 6 6 6 7 7 7 7
  line L207 (161.6301, 51.7) -> (161.6301, 38.1)
  spline S146 degree 3 poles (161.4301, 37.9) (161.5405, 37.9) (161.6301, 37.9895) (161.6301, 38.1) knots 4 4 4 4 5 5 5 5
  line L208 (161.4301, 37.9) -> (147.8301, 37.9)
  spline S147 degree 3 poles (147.6301, 38.1) (147.6301, 37.9895) (147.7197, 37.9) (147.8301, 37.9) knots 2 2 2 2 3 3 3 3
  line L209 (147.6301, 38.1) -> (147.6301, 51.7)
  spline S148 degree 3 poles (147.8301, 51.9) (147.7197, 51.9) (147.6301, 51.8104) (147.6301, 51.7) knots 0 0 0 0 1 1 1 1
  line L210 (147.8301, 51.9) -> (161.4301, 51.9)
  line L211 (272.2807, 51.63) -> (272.2807, 52.88)
  line L212 (272.2807, 52.88) -> (275.2807, 52.88)
  line L213 (275.2807, 52.88) -> (275.2807, 51.63)
  line L214 (275.2807, 51.63) -> (277.1057, 51.63)
  line L215 (277.1057, 51.63) -> (277.1057, 45.43)
  line L216 (277.1057, 45.43) -> (277.9307, 45.43)
  line L217 (277.9307, 45.43) -> (277.9307, 42.42)
  line L218 (277.9307, 42.42) -> (277.1057, 42.42)
  line L219 (277.1057, 42.42) -> (277.1057, 39.42)
  line L220 (277.1057, 39.42) -> (270.4557, 39.42)
  line L221 (270.4557, 39.42) -> (270.4557, 41.92)
  line L222 (270.4557, 41.92) -> (268.78, 41.92)
  line L223 (268.78, 41.92) -> (268.78, 38.1)
  spline S149 degree 3 poles (268.5802, 37.9) (268.6906, 37.9) (268.78, 37.9895) (268.78, 38.1) knots 25 25 25 25 26 26 26 26
  line L224 (268.5802, 37.9) -> (254.9801, 37.9)
  spline S150 degree 3 poles (254.7801, 38.1) (254.7801, 37.9895) (254.8695, 37.9) (254.9801, 37.9) knots 23 23 23 23 24 24 24 24
  line L225 (254.7801, 38.1) -> (254.7801, 41.92)
  line L226 (254.7801, 41.92) -> (253.1046, 41.92)
  line L227 (253.1046, 41.92) -> (253.1046, 39.42)
  line L228 (253.1046, 39.42) -> (246.4547, 39.42)
  line L229 (246.4547, 39.42) -> (246.4547, 42.42)
  line L230 (246.4547, 42.42) -> (245.6298, 42.42)
  line L231 (245.6298, 42.42) -> (245.6298, 45.43)
  line L232 (245.6298, 45.43) -> (246.4547, 45.43)
  line L233 (246.4547, 45.43) -> (246.4547, 51.63)
  line L234 (246.4547, 51.63) -> (248.2798, 51.63)
  line L235 (248.2798, 51.63) -> (248.2798, 52.88)
  line L236 (248.2798, 52.88) -> (251.2798, 52.88)
  line L237 (251.2798, 52.88) -> (251.2798, 51.63)
  line L238 (251.2798, 51.63) -> (253.1046, 51.63)
  line L239 (253.1046, 51.63) -> (253.1046, 49.13)
  line L240 (253.1046, 49.13) -> (254.7801, 49.13)
  line L241 (254.7801, 49.13) -> (254.7801, 51.7)
  spline S151 degree 3 poles (254.9801, 51.9) (254.8695, 51.9) (254.7801, 51.8104) (254.7801, 51.7) knots 5 5 5 5 6 6 6 6
  line L242 (254.9801, 51.9) -> (268.5802, 51.9)
  spline S152 degree 3 poles (268.78, 51.7) (268.78, 51.8104) (268.6906, 51.9) (268.5802, 51.9) knots 3 3 3 3 4 4 4 4
  line L243 (268.78, 51.7) -> (268.78, 49.13)
  line L244 (268.78, 49.13) -> (270.4557, 49.13)
  line L245 (270.4557, 49.13) -> (270.4557, 51.63)
  line L246 (270.4557, 51.63) -> (272.2807, 51.63)
  spline S153 degree 3 poles (299.55, 18.85) (299.6604, 18.85) (299.75, 18.9395) (299.75, 19.05) knots 6 6 6 6 7 7 7 7
  line L247 (299.55, 18.85) -> (285.95, 18.85)
  spline S154 degree 3 poles (285.75, 19.05) (285.75, 18.9395) (285.8396, 18.85) (285.95, 18.85) knots 4 4 4 4 5 5 5 5
  line L248 (285.75, 19.05) -> (285.75, 32.65)
  spline S155 degree 3 poles (285.95, 32.85) (285.8396, 32.85) (285.75, 32.7604) (285.75, 32.65) knots 2 2 2 2 3 3 3 3
  line L249 (285.95, 32.85) -> (299.55, 32.85)
  spline S156 degree 3 poles (299.75, 32.65) (299.75, 32.7604) (299.6604, 32.85) (299.55, 32.85) knots 0 0 0 0 1 1 1 1
  line L250 (299.75, 32.65) -> (299.75, 19.05)
  spline S157 degree 3 poles (299.55, 56.95) (299.6604, 56.95) (299.75, 57.0395) (299.75, 57.15) knots 6 6 6 6 7 7 7 7
  line L251 (299.55, 56.95) -> (285.95, 56.95)
  spline S158 degree 3 poles (285.75, 57.15) (285.75, 57.0395) (285.8396, 56.95) (285.95, 56.95) knots 4 4 4 4 5 5 5 5
  line L252 (285.75, 57.15) -> (285.75, 70.75)
  spline S159 degree 3 poles (285.95, 70.95) (285.8396, 70.95) (285.75, 70.8604) (285.75, 70.75) knots 2 2 2 2 3 3 3 3
  line L253 (285.95, 70.95) -> (299.55, 70.95)
  spline S160 degree 3 poles (299.75, 70.75) (299.75, 70.8604) (299.6604, 70.95) (299.55, 70.95) knots 0 0 0 0 1 1 1 1
  line L254 (299.75, 70.75) -> (299.75, 57.15)
  spline S161 degree 3 poles (299.55, 76) (299.6604, 76) (299.75, 76.0895) (299.75, 76.2) knots 6 6 6 6 7 7 7 7
  line L255 (299.55, 76) -> (285.95, 76)
  spline S162 degree 3 poles (285.75, 76.2) (285.75, 76.0895) (285.8396, 76) (285.95, 76) knots 4 4 4 4 5 5 5 5
  line L256 (285.75, 76.2) -> (285.75, 89.8)
  spline S163 degree 3 poles (285.95, 90) (285.8396, 90) (285.75, 89.9104) (285.75, 89.8) knots 2 2 2 2 3 3 3 3
  line L257 (285.95, 90) -> (299.55, 90)
  spline S164 degree 3 poles (299.75, 89.8) (299.75, 89.9104) (299.6604, 90) (299.55, 90) knots 0 0 0 0 1 1 1 1
  line L258 (299.75, 89.8) -> (299.75, 76.2)
  spline S165 degree 3 poles (299.55, 37.9) (299.6604, 37.9) (299.75, 37.9895) (299.75, 38.1) knots 6 6 6 6 7 7 7 7
  line L259 (299.55, 37.9) -> (285.95, 37.9)
  spline S166 degree 3 poles (285.75, 38.1) (285.75, 37.9895) (285.8396, 37.9) (285.95, 37.9) knots 4 4 4 4 5 5 5 5
  line L260 (285.75, 38.1) -> (285.75, 51.7)
  spline S167 degree 3 poles (285.95, 51.9) (285.8396, 51.9) (285.75, 51.8104) (285.75, 51.7) knots 2 2 2 2 3 3 3 3
  line L261 (285.95, 51.9) -> (299.55, 51.9)
  spline S168 degree 3 poles (299.75, 51.7) (299.75, 51.8104) (299.6604, 51.9) (299.55, 51.9) knots 0 0 0 0 1 1 1 1
  line L262 (299.75, 51.7) -> (299.75, 38.1)
  spline S169 degree 3 poles (228.8, 13.8) (228.6896, 13.8) (228.6, 13.7104) (228.6, 13.6) knots 6 6 6 6 7 7 7 7
  line L263 (228.8, 13.8) -> (242.4, 13.8)
  spline S170 degree 3 poles (242.6, 13.6) (242.6, 13.7104) (242.5104, 13.8) (242.4, 13.8) knots 4 4 4 4 5 5 5 5
  line L264 (242.6, 13.6) -> (242.6, 0)
  spline S171 degree 3 poles (242.4, -0.2) (242.5104, -0.2) (242.6, -0.1105) (242.6, 0) knots 2 2 2 2 3 3 3 3
  line L265 (242.4, -0.2) -> (228.8, -0.2)
  spline S172 degree 3 poles (228.6, 0) (228.6, -0.1105) (228.6896, -0.2) (228.8, -0.2) knots 0 0 0 0 1 1 1 1
  line L266 (228.6, 0) -> (228.6, 13.6)
  spline S173 degree 3 poles (252.13, 32.65) (252.13, 32.7604) (252.0406, 32.85) (251.93, 32.85) knots 6 6 6 6 7 7 7 7
  line L267 (252.13, 32.65) -> (252.13, 19.05)
  spline S174 degree 3 poles (251.93, 18.85) (252.0406, 18.85) (252.13, 18.9395) (252.13, 19.05) knots 4 4 4 4 5 5 5 5
  line L268 (251.93, 18.85) -> (238.3302, 18.85)
  spline S175 degree 3 poles (238.13, 19.05) (238.13, 18.9395) (238.2196, 18.85) (238.3302, 18.85) knots 2 2 2 2 3 3 3 3
  line L269 (238.13, 19.05) -> (238.13, 32.65)
  spline S176 degree 3 poles (238.3302, 32.85) (238.2196, 32.85) (238.13, 32.7604) (238.13, 32.65) knots 0 0 0 0 1 1 1 1
  line L270 (238.3302, 32.85) -> (251.93, 32.85)
  line L271 (262.1401, 32.85) -> (275.7401, 32.85)
  spline S177 degree 3 poles (275.9401, 32.65) (275.9401, 32.7604) (275.8505, 32.85) (275.7401, 32.85) knots 5 5 5 5 6 6 6 6
  line L272 (275.9401, 32.65) -> (275.9401, 19.05)
  spline S178 degree 3 poles (275.7401, 18.85) (275.8505, 18.85) (275.9401, 18.9395) (275.9401, 19.05) knots 3 3 3 3 4 4 4 4
  line L273 (275.7401, 18.85) -> (262.1401, 18.85)
  spline S179 degree 3 poles (261.9401, 19.05) (261.9401, 18.9395) (262.0297, 18.85) (262.1401, 18.85) knots 1 1 1 1 2 2 2 2
  line L274 (261.9401, 19.05) -> (261.9401, 32.65)
  spline S180 degree 3 poles (262.1401, 32.85) (262.0297, 32.85) (261.9401, 32.7604) (261.9401, 32.65) knots 7 7 7 7 8 8 8 8